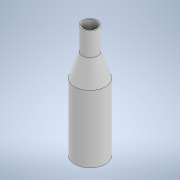
# Autodesk Inventor part: Pièce35
Saved by Autodesk Inventor 2020 (Build 240168000, 168)
## iProperties
Created: 2023-09-29
Part Number: Pièce35
Material: Générique
Document SubType Name: Modeling
Designer: Admin
Density: 1 g/cm^3
Appearance: Par défaut
Author: Admin
Autodesk Inventor part; units mm, degrees
ref_plane "YZ Plane" through (0, 0, 0) normal (1, 0, 0) x (0, 1, 0)
ref_plane "XZ Plane" through (0, 0, 0) normal (0, 1, 0) x (-1, 0, 0)
ref_plane "XY Plane" through (0, 0, 0) normal (0, 0, 1) x (1, 0, 0)
sketch "Esquisse3" plane through (0, 0, 0) normal (0, 0, 1) x (1, 0, 0)
  line L0 (0, 0) -> (25.2376, 0)
  line L1 (25.2376, 0) -> (25.2376, 58.756)
  line L2 (25.2376, 58.756) -> (25.2376, 118.9226)
  line L3 (25.2376, 118.9226) -> (11.8572, 160.0383)
  line L4 (11.8572, 160.0383) -> (11.8572, 201.5839)
  line L5 (0, 244.1266) -> (0, -47.634)
  line L6 (13.8572, 201.5839) -> (13.8572, 160.3556)
  line L7 (13.8572, 160.3556) -> (27.2376, 119.2398)
  line L8 (27.2376, 119.2398) -> (27.2376, 58.756)
  line L9 (27.2376, 58.756) -> (27.2376, -2)
  line L10 (27.2376, -2) -> (0, -2)
  line L11 (11.8572, 201.5839) -> (13.8572, 201.5839)
  line L12 (25.2376, 0) -> (27.2376, 0)
  dimension "d2" = 58.756
  dimension "d3" = 90
  dimension "d4" = 2
  constraints: 26 end point, 3 perpendicular, 2 horizontal, 2 parallel, 2 point on line, 1 vertical, 4 other
  measures "d2" distance of L0.end L1.end
  measures "d3" angle of L1 L0
  measures "d4" distance between parallel lines of L3 L7
revolve "Révolution1" add sketch "Esquisse3" angle 360 about axis through (0, 244.1266, 0) along (0, -1, 0) contours L1 L2 L3 L4 L11 L6 L7 L8 L9 L12
